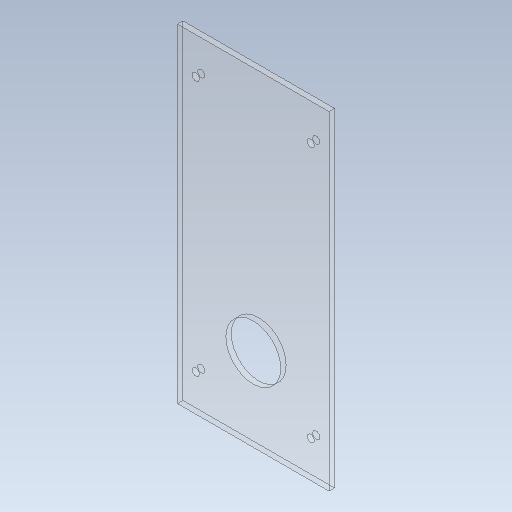
# Autodesk Inventor part: BaseC_3
Saved by Autodesk Inventor 2021.1 (Build 251245010, 245A)
## iProperties
Created: 2023-10-20
Part Number: BaseC_3
Material: PMMA Plastic
Document SubType Name: Modeling
Designer: user
Density: 1.188 g/cm^3
Appearance: Polycarbonate - Clear
Author: user
Autodesk Inventor part; units mm, degrees
ref_plane "YZ Plane" through (0, 0, 0) normal (1, 0, 0) x (0, 1, 0)
ref_plane "XZ Plane" through (0, 0, 0) normal (0, 1, 0) x (-1, 0, 0)
ref_plane "XY Plane" through (0, 0, 0) normal (0, 0, 1) x (1, 0, 0)
sketch "Sketch1" plane through (0, 0, 0) normal (0, 0, 1) x (1, 0, 0)
  line L0 (83, 0) -> (83, 180)
  line L1 (83, 180) -> (0, 180)
  line L2 (0, 180) -> (0, 0)
  circle A0 centre (41.5, 45) radius 15
  line L3 (0, 0) -> (83, 0)
  line L4 (10, 171.8151) -> (10, 9.9445)
  line L5 (73, 174.9264) -> (73, 13.0559)
  circle A1 centre (10, 160) radius 2
  circle A2 centre (73, 160) radius 2
  circle A3 centre (10, 20) radius 2
  circle A4 centre (73, 20) radius 2
  dimension "d0" = 83
  dimension "d1" = 180
  dimension "d4" = 30
  dimension "d5" = 41.5
  dimension "d10" = 10
  dimension "d11" = 10
  dimension "d12" = 4
  dimension "d13" = 20
  dimension "d14" = 20
  dimension "d15" = 20
  dimension "d16" = 20
  dimension "d17" = 4
  dimension "d18" = 4
  dimension "d19" = 4
  constraints: 12 end point, 5 centre point, 4 point on line, 2 parallel, 2 vertical, 1 horizontal, 1 perpendicular
  measures "d0" distance of L1.end L0.end
  measures "d1" distance of L0.end L0.start
  measures "d4" diameter of A0
  measures "d5" distance from line of L0 A0.centre
  measures "d10" distance between parallel lines of L0 L5
  measures "d11" distance between parallel lines of L2 L4
  measures "d12" diameter of A1
  measures "d13" distance from line of L1 A1.centre
  measures "d14" distance from line of L1 A2.centre
  measures "d15" distance from line of L3 A4.centre
  measures "d16" distance from line of L3 A3.centre
  measures "d17" diameter of A2
  measures "d18" diameter of A3
  measures "d19" diameter of A4
extrude "Extrusion1" add sketch "Sketch1" along normal blind 3
equation "\"d5\" = 0.5 * d0"
equation "\"d11\" = d10"
equation "\"d14\" = d13"
equation "\"d15\" = d13"
equation "\"d16\" = d13"
equation "\"d17\" = d12"
equation "\"d18\" = d12"
equation "\"d19\" = d18"
equation "\"d6\" = 0.25 * d1"
body "Solid1"
